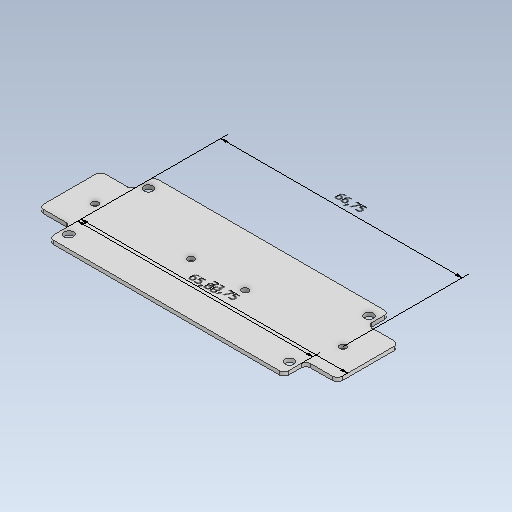
# Autodesk Inventor part: Interstage B1
Saved by Autodesk Inventor 2020.3 (Build 243373000, 373)
## iProperties
Created: 2020-05-18
Part Number: Interstage B1
Material: Genérico
Document SubType Name: Modeling
Designer: javic
Density: 1 g/cm^3
Appearance: Valor por defecto
Author: javic
Autodesk Inventor part; units mm, degrees
ref_plane "YZ Plane" through (0, 0, 0) normal (1, 0, 0) x (0, 1, 0)
ref_plane "XZ Plane" through (0, 0, 0) normal (0, 1, 0) x (-1, 0, 0)
ref_plane "XY Plane" through (0, 0, 0) normal (0, 0, 1) x (1, 0, 0)
sketch "Boceto1" plane through (0, 0, 0) normal (0, 1, 0) x (-1, 0, 0)
  arc A0 (-10.02, 7.27) -> (-8.75, 6) centre (-8.75, 7.27) ccw
  line L0 (-8.75, 6) -> (-2.54, 6)
  arc A1 (-1.27, 4.73) -> (-2.54, 6) centre (-2.54, 4.73) ccw
  line L1 (-1.27, 4.73) -> (-1.27, 1.27)
  arc A2 (-1.27, 1.27) -> (0, 0) centre (0, 1.27) ccw
  line L2 (0, 0) -> (62.46, 0)
  arc A3 (62.46, 0) -> (63.73, 1.27) centre (62.46, 1.27) ccw
  line L3 (63.73, 1.27) -> (63.73, 4.73)
  arc A4 (65, 6) -> (63.73, 4.73) centre (65, 4.73) ccw
  line L4 (65, 6) -> (71.21, 6)
  arc A5 (71.21, 6) -> (72.48, 7.27) centre (71.21, 7.27) ccw
  line L5 (72.48, 7.27) -> (72.48, 21.73)
  arc A6 (72.48, 21.73) -> (71.21, 23) centre (71.21, 21.73) ccw
  line L6 (71.21, 23) -> (65, 23)
  arc A7 (63.73, 24.27) -> (65, 23) centre (65, 24.27) ccw
  line L7 (63.73, 24.27) -> (63.73, 27.73)
  arc A8 (63.73, 27.73) -> (62.46, 29) centre (62.46, 27.73) ccw
  line L8 (62.46, 29) -> (0, 29)
  arc A9 (0, 29) -> (-1.27, 27.73) centre (0, 27.73) ccw
  line L9 (-1.27, 27.73) -> (-1.27, 24.27)
  arc A10 (-2.54, 23) -> (-1.27, 24.27) centre (-2.54, 24.27) ccw
  line L10 (-2.54, 23) -> (-8.75, 23)
  arc A11 (-8.75, 23) -> (-10.02, 21.73) centre (-8.75, 21.73) ccw
  line L11 (-10.02, 21.73) -> (-10.02, 7.27)
  circle A12 centre (61.755, 25.475) radius 1.25
  circle A13 centre (0.755, 3.475) radius 1.25
  circle A14 centre (0.755, 25.475) radius 1.25
  circle A15 centre (61.755, 3.475) radius 1.25
  circle A16 centre (38.98, 14.5) radius 0.9
  circle A17 centre (23.98, 14.5) radius 0.9
  point P0 (0, 0)
  constraints: 27 tangent, 24 end point, 24 point on circle, 18 centre point, 15 equal radius, 4 parallel, 4 perpendicular
extrude "Extrusión1" add sketch "Boceto1" along normal blind 1.04
sketch "Boceto2" plane through (0, 1.04, 0) normal (0, 1, 0) x (1, 0, 0)
  circle A0 centre (-65.48, -14.5) radius 0.9
  circle A1 centre (3.02, -14.5) radius 0.9
  line L0 (-71.21, -23) -> (-65, -23) projected
  line L1 (-72.48, -7.27) -> (-72.48, -21.73) projected
  line L2 (2.54, -23) -> (8.75, -23) projected
  line L3 (10.02, -21.73) -> (10.02, -7.27) projected
  point P0 (0, 0)
  dimension "d2" = 1.8
  dimension "d3" = 1.8
  dimension "d4" = 8.5
  dimension "d5" = 7
  dimension "d6" = 8.5
  dimension "d7" = 7
  constraints: 2 centre point
  measures "d2" diameter of A0
  measures "d3" diameter of A1
  measures "d4" distance from line of L0 A0.centre
  measures "d5" distance from line of L1 A0.centre
  measures "d6" distance from line of L2 A1.centre
  measures "d7" distance from line of L3 A1.centre
hole "Agujero1" at (-65.48, 1.04, 14.5) at (3.02, 1.04, 14.5) direction (0, -1, 0) diameter 1.8 end through all
